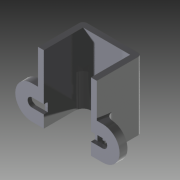
# Autodesk Inventor part: Pololu Micro Metal Gearmotor Bracket Extended
Saved by Autodesk Inventor 2013 SP2 (Build 170200200, 200)
## iProperties
Created: 2014-04-15
Part Number: Pololu Micro Metal Gearmotor Bracket Extended
Material: Generic
Document SubType Name: Modeling
Designer: Kevin
Density: 1 g/cm^3
Author: Kevin
Autodesk Inventor part; units mm, degrees
ref_plane "YZ Plane" through (0, 0, 0) normal (1, 0, 0) x (0, 1, 0)
ref_plane "XZ Plane" through (0, 0, 0) normal (0, 1, 0) x (-1, 0, 0)
ref_plane "XY Plane" through (0, 0, 0) normal (0, 0, 1) x (1, 0, 0)
sketch "Sketch1" plane through (0, 0, 0) normal (0, 0, 1) x (1, 0, 0)
  line L0 (7.5, 0) -> (7.5, 11.5)
  line L1 (7.5, 11.5) -> (0, 11.5)
  line L2 (0, 11.5) -> (0, 10)
  line L3 (6, 5) -> (6, 0)
  line L4 (6, 5) -> (6, 8)
  line L5 (0, 10) -> (4, 10)
  arc A0 (6, 8) -> (4, 10) centre (4, 8) ccw
  line L6 (6, 0) -> (7.5, 0)
  point P0 (0, 0)
  dimension "d0" = 7.5
  dimension "d1" = 11.5
  dimension "d6" = 2
  constraints: 14 end point, 4 perpendicular, 2 parallel, 2 point on circle, 2 tangent, 1 centre point, 1 horizontal
  measures "d0" distance of L1.end L0.end
  measures "d1" distance of L0.end L0.start
  measures "d6" radius of A0
extrude "Extrusion1" add sketch "Sketch1" along normal blind 17.3
sketch "Sketch2" plane through (0, 0, 17.3) normal (0, 0, 1) x (1, 0, 0)
  line L0 (7.5, 11.5) -> (0, 11.5) projected
  arc A0 (6, 8) -> (4, 10) centre (4, 8) ccw projected
  line L1 (7.5, 11.5) -> (6, 11.5)
  line L2 (6, 11.5) -> (6, 10)
  line L3 (6, 10) -> (4, 10)
  line L4 (4, 10) -> (4, 8)
  line L5 (4, 8) -> (6, 8)
  line L6 (6, 8) -> (6, 10)
  point P0 (0, 0)
  constraints: 12 end point, 2 parallel, 2 perpendicular, 1 horizontal, 1 point on line
extrude "Extrusion2" cut sketch "Sketch2" against normal blind 9
fillet "Fillet1" radius 1 1 edges at (7.5, 11.5, 8.65)
sketch "Sketch3" plane through (7.5, 0, 17.3) normal (1, 0, 0) x (0, 0, -1)
  line L0 (17.3, 0) -> (8.8, 0)
  line L1 (8.8, 0) -> (8.8, 2)
  line L2 (8.8, 2) -> (17.3, 2)
  line L3 (17.3, 2) -> (17.3, 0)
  dimension "d12" = 8.5
  dimension "d13" = 2
  constraints: 8 end point, 2 parallel, 1 horizontal, 1 perpendicular
  measures "d12" distance of L1.end L2.end
  measures "d13" distance of L0.end L1.end
extrude "Extrusion3" add sketch "Sketch3" along normal blind 5.8
fillet "Fillet2" radius 4.25 1 edges at (13.3, 1, 0)
fillet "Fillet3" radius 4.25 1 edges at (13.3, 1, 8.5)
sketch "Sketch4" plane through (7.5, 2, 8.5) normal (0, 1, 0) x (1, 0, 0)
  arc A0 (1.55, 0) -> (1.55, 8.5) centre (1.55, 4.25) ccw projected
  line L0 (3.9313, 2.8752) -> (1.55, 1.5004)
  line L1 (1.55, 1.5004) -> (-0.8313, 2.8752)
  line L2 (-0.8313, 2.8752) -> (-0.8313, 5.6248)
  line L3 (-0.8313, 5.6248) -> (1.55, 6.9996)
  line L4 (1.55, 6.9996) -> (3.9312, 5.6248)
  line L5 (3.9312, 5.6248) -> (3.9313, 2.8752)
  point P0 (-7.5, 8.5)
  constraints: 12 end point, 1 coincident, 13 other
extrude "Extrusion4" cut sketch "Sketch4" against normal blind 1
sketch "Sketch5" plane through (6, 0, 0) normal (-1, 0, 0) x (0, 0, 1)
  line L0 (0, 0) -> (17.3, 0) projected
  line L1 (0, 0) -> (4.25, 0)
  line L2 (4.25, 0) -> (3.1197, 0)
  line L3 (3.1197, 0) -> (3.1197, 1)
  line L4 (3.1197, 1) -> (4.25, 1)
  line L5 (4.25, 1) -> (4.25, 0)
  line L6 (4.25, 0) -> (5.3803, 0)
  line L7 (5.3803, 0) -> (5.3803, 1)
  line L8 (5.3803, 1) -> (4.25, 1)
  line L9 (4.25, 1) -> (4.25, 0)
  dimension "d22" = 4.25
  dimension "d23" = 1.1303
  dimension "d24" = 1
  dimension "d25" = 1.1303
  constraints: 18 end point, 4 parallel, 2 horizontal, 2 perpendicular, 1 point on line
  measures "d22" distance of L0.start L1.end
  measures "d23" distance of L3.end L4.end
  measures "d24" distance of L2.end L3.end
  measures "d25" distance of L8.end L7.end
extrude "Extrusion5" cut sketch "Sketch5" against normal blind 3
sketch "Sketch6" plane through (7.5, 1, 8.5) normal (0, 1, 0) x (1, 0, 0)
  line L0 (1.5, 5.3803) -> (1.5, 3.1197) projected
  circle A0 centre (1.5, 4.25) radius 1.1303
  point P0 (-7.5, 8.5)
  constraints: 1 midpoint, 1 vertical alignment, 2 other
extrude "Extrusion6" cut sketch "Sketch6" against normal blind 1
fillet "Fillet4" radius 2 1 edges at (7.5, 2, 1.1976)
fillet "Fillet5" radius 2 1 edges at (7.5, 2, 7.3024)
mirror "Mirror1" about plane through (0, 11.5, 0) normal (-1, 0, 0) of "Extrusion1", "Extrusion2", "Fillet1", "Extrusion3", "Fillet2", "Fillet3", "Extrusion4", "Extrusion5", "Extrusion6", "Fillet4", "Fillet5"
body "Solid1"
